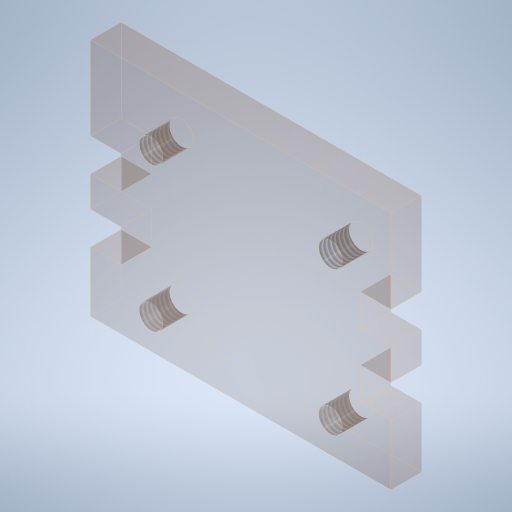
# Autodesk Inventor part: caster wheel mounter
Saved by Autodesk Inventor 2023.2 (Build 272271000, 271)
## iProperties
Created: 2024-08-13
Part Number: caster wheel mounter
Material: Polycarbonate, Clear
Document SubType Name: Modeling
Designer: PC
Density: 1.2 g/cm^3
Appearance: Polycarbonate - Smoked
Author: PC
Autodesk Inventor part; units mm, degrees
ref_plane "YZ Plane" through (0, 0, 0) normal (1, 0, 0) x (0, 1, 0)
ref_plane "XZ Plane" through (0, 0, 0) normal (0, 1, 0) x (-1, 0, 0)
ref_plane "XY Plane" through (0, 0, 0) normal (0, 0, 1) x (1, 0, 0)
sketch "Sketch1" plane through (0, 0, 0) normal (0, 0, 1) x (1, 0, 0)
  line L0 (20.01, -20) -> (-20.01, -20)
  line L1 (-20.01, -20) -> (-20.01, 20)
  line L2 (-20.01, 20) -> (20.01, 20)
  line L3 (20.01, 20) -> (20.01, -20)
  line L4 (20.01, -20) -> (-20.01, 20) construction
  line L5 (-20.01, -20) -> (20.01, 20) construction
  line L6 (-20.01, 20) -> (-25.11, 20)
  line L7 (-25.11, 20) -> (-25.11, -20)
  line L8 (-25.11, -20) -> (-20.01, -20)
  line L9 (-20.01, -20) -> (-20.01, 20)
  line L10 (20.01, 20) -> (25.11, 20)
  line L11 (25.11, 20) -> (25.11, -20)
  line L12 (25.11, -20) -> (20.01, -20)
  line L13 (20.01, -20) -> (20.01, 20)
  point P0 (0, 0)
  point P1 (20.01, -20)
  dimension "d0" = 40.02
  dimension "d1" = 40
  dimension "d2" = 5.1
  dimension "d3" = 5.1
  constraints: 28 end point, 6 parallel, 3 horizontal, 3 perpendicular, 2 midpoint, 1 point on line
  measures "d0" distance of L1.end L2.end
  measures "d1" distance of L0.end L1.end
  measures "d2" distance of L8.end L7.end
  measures "d3" distance of L11.end L12.end
extrude "Extrusion1" add sketch "Sketch1" along normal blind 5.1 contours L0 L1 L2 L3
sketch "Sketch3" plane through (0, 0, 0) normal (0, 0, -1) x (-1, 0, 0)
  circle A0 centre (15, -15) radius 2
  circle A1 centre (-15, -15) radius 2
  circle A2 centre (15, 9.06) radius 2
  circle A3 centre (-15, 9.06) radius 2
  point P0 (0, 0)
  dimension "d8" = 4
  dimension "d9" = 4
  dimension "d10" = 4
  dimension "d11" = 4
  dimension "d12" = 15
  dimension "d14" = 15
  dimension "d16" = 15
  dimension "d17" = 15
  dimension "d18" = 15
  dimension "d19" = 15
  dimension "d30" = 24.06
  dimension "d31" = 24.06
  constraints: 4 centre point
  measures "d8" diameter of A0
  measures "d9" diameter of A1
  measures "d10" diameter of A2
  measures "d11" diameter of A3
  measures "d12" horizontal distance of point (0, 0) A0.centre
  measures "d14" horizontal distance of point (0, 0) A1.centre
  measures "d16" horizontal distance of point (0, 0) A3.centre
  measures "d17" horizontal distance of A2.centre point (0, 0)
  measures "d18" horizontal distance of point (0, 0) A0.centre
  measures "d19" horizontal distance of point (0, 0) A1.centre
  measures "d30" distance of A0.centre A2.centre
  measures "d31" distance of A3.centre A1.centre
extrude "Extrusion3" cut sketch "Sketch3" against normal blind 10
thread "Thread1" size "M4x0.7" class "6H" standard "ANSI Metric M Profile" length 150
thread "Thread2" size "M4x0.7" class "6H" standard "ANSI Metric M Profile" length 150
thread "Thread3" size "M4x0.7" class "6H" standard "ANSI Metric M Profile" length 150
thread "Thread4" size "M4x0.7" class "6H" standard "ANSI Metric M Profile" length 150
sketch "Sketch4" plane through (0, 0, 0) normal (0, 0, -1) x (-1, 0, 0)
  line L0 (20.01, 20) -> (20.01, -20) projected
  line L1 (20.01, -10) -> (14.91, -10)
  line L2 (14.91, -10) -> (14.91, -4.5)
  line L3 (14.91, -4.5) -> (20.01, -4.5)
  line L4 (20.01, -4.5) -> (20.01, -10)
  line L5 (20.01, -20) -> (-20.01, -20) projected
  line L6 (20.01, 0.6) -> (14.91, 0.6)
  line L7 (14.91, 0.6) -> (14.91, 6.1)
  line L8 (14.91, 6.1) -> (20.01, 6.1)
  line L9 (20.01, 6.1) -> (20.01, 0.6)
  line L10 (-20.01, 20) -> (20.01, 20) projected
  line L11 (0, 0) -> (0, -7.4) construction
  line L12 (-20.01, -10) -> (-14.91, -10)
  line L13 (-14.91, -10) -> (-14.91, -4.5)
  line L14 (-14.91, -4.5) -> (-20.01, -4.5)
  line L15 (-20.01, -4.5) -> (-20.01, -10)
  line L16 (-20.01, 0.6) -> (-14.91, 0.6)
  line L17 (-14.91, 0.6) -> (-14.91, 6.1)
  line L18 (-14.91, 6.1) -> (-20.01, 6.1)
  line L19 (-20.01, 6.1) -> (-20.01, 0.6)
  dimension "d32" = 5.1
  dimension "d33" = 5.5
  dimension "d34" = 10
  dimension "d35" = 5.1
  dimension "d36" = 5.5
  dimension "d37" = 13.9
  constraints: 34 end point, 8 symmetric about line, 4 parallel, 2 horizontal, 2 perpendicular, 2 point on line, 1 vertical
  measures "d32" distance of L2.end L3.end
  measures "d33" distance of L1.end L2.end
  measures "d34" distance between parallel lines of L5 L1
  measures "d35" distance of L7.end L8.end
  measures "d36" distance of L6.end L7.end
  measures "d37" distance between parallel lines of L10 L8
extrude "Extrusion4" cut sketch "Sketch4" against normal blind 10
sketch "Sketch5" plane through (-20.01, -20, 0) normal (-1, 0, 0) x (0, 0, 1)
  line L0 (5.1, 10) -> (0, 10) projected
  line L1 (0, 10) -> (0, 0) projected
  line L2 (0, 0) -> (5.1, 0) projected
  line L3 (5.1, 10) -> (5.1, 0) projected
  line L4 (5.1, 20.6) -> (0, 20.6) projected
  line L5 (0, 20.6) -> (0, 15.5) projected
  line L6 (0, 15.5) -> (5.1, 15.5) projected
  line L7 (5.1, 20.6) -> (5.1, 15.5) projected
  line L8 (0, 26.1) -> (5.1, 26.1) projected
  line L9 (5.1, 40) -> (5.1, 26.1) projected
  line L10 (0, 40) -> (5.1, 40) projected
  line L11 (0, 40) -> (0, 26.1) projected
  point P0 (0, 20)
extrude "Extrusion5" add sketch "Sketch5" along normal blind 5.1
sketch "Sketch6" plane through (20.01, -20, 5.1) normal (1, 0, 0) x (0, 0, -1)
  line L0 (5.1, 10) -> (0, 10) projected
  line L1 (0, 0) -> (0, 10) projected
  line L2 (5.1, 0) -> (0, 0) projected
  line L3 (5.1, 0) -> (5.1, 10) projected
  line L4 (0, 15.5) -> (5.1, 15.5) projected
  line L5 (5.1, 15.5) -> (5.1, 20.6) projected
  line L6 (5.1, 20.6) -> (0, 20.6) projected
  line L7 (0, 15.5) -> (0, 20.6) projected
  line L8 (5.1, 31.06) -> (0, 31.06) projected
  line L9 (0, 26.1) -> (5.1, 26.1) projected
  line L10 (5.1, 26.1) -> (5.1, 40) projected
  line L11 (5.1, 40) -> (0, 40) projected
  line L12 (0, 26.1) -> (0, 40) projected
  point P0 (5.1, 20)
extrude "Extrusion6" add sketch "Sketch6" along normal blind 5.1
sketch "Sketch7" plane through (0, 0, 0) normal (0, 0, -1) x (-1, 0, 0)
  line L0 (14.91, -10) -> (14.91, -4.5) projected
  line L1 (14.91, -10) -> (25.11, -10) projected
  line L2 (14.91, -4.5) -> (20.01, -4.5)
  line L3 (20.01, -4.5) -> (20.01, -10)
  line L4 (20.01, -10) -> (14.91, -10)
  line L5 (14.91, -10) -> (14.91, -4.5)
  line L6 (14.91, 0.6) -> (14.91, 6.1) projected
  line L7 (14.91, 6.1) -> (25.11, 6.1) projected
  line L8 (14.91, 0.6) -> (20.01, 0.6)
  line L9 (20.01, 0.6) -> (20.01, 6.1)
  line L10 (20.01, 6.1) -> (14.91, 6.1)
  line L11 (14.91, 6.1) -> (14.91, 0.6)
  line L12 (-14.91, -10) -> (-25.11, -10) projected
  line L13 (-14.91, -4.5) -> (-25.11, -4.5) projected
  line L14 (-14.91, -10) -> (-20.01, -10)
  line L15 (-20.01, -10) -> (-20.01, -4.5)
  line L16 (-20.01, -4.5) -> (-14.91, -4.5)
  line L17 (-14.91, -4.5) -> (-14.91, -10)
  line L18 (-14.91, 6.1) -> (-14.91, 0.6) projected
  line L19 (-14.91, 0.6) -> (-25.11, 0.6) projected
  line L20 (-14.91, 6.1) -> (-20.01, 6.1)
  line L21 (-20.01, 6.1) -> (-20.01, 0.6)
  line L22 (-20.01, 0.6) -> (-14.91, 0.6)
  line L23 (-14.91, 0.6) -> (-14.91, 6.1)
  point P0 (0, 0)
  dimension "d44" = 5.1
  dimension "d45" = 5.1
  constraints: 32 end point, 8 parallel, 4 horizontal, 4 midpoint, 4 perpendicular
  measures "d44" distance of L3.end L4.end
  measures "d45" distance of L15.end L16.end
extrude "Extrusion7" add sketch "Sketch7" against normal blind 5.1
body "Solid1"
